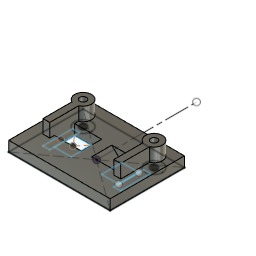
sensor_base (Autodesk Fusion 360 design; units mm, degrees)
Autodesk Fusion 360 part; units mm, degrees
sketch "Schizzo1" plane through (0, 0, 0) normal (0, 0, 1) x (1, 0, 0)
  line L0 (15, -11) -> (-15, -11)
  line L1 (-15, -11) -> (-15, 11)
  line L2 (-15, 11) -> (15, 11)
  line L3 (15, 11) -> (15, -11)
  line L4 (15, -11) -> (-15, 11) construction
  line L5 (-15, -11) -> (15, 11) construction
  circle A0 centre (-10.5, 6.5) radius 1
  line L6 (0, 0) -> (0, 29.5876)
  circle A1 centre (10.5, 6.5) radius 1
  line L7 (-4.5, -3) -> (-9.5, -3)
  line L8 (-9.5, -3) -> (-9.5, 3)
  line L9 (-9.5, 3) -> (-4.5, 3)
  line L10 (-4.5, 3) -> (-4.5, -3)
  line L11 (-4.5, -3) -> (-9.5, 3) construction
  line L12 (-9.5, -3) -> (-4.5, 3) construction
  line L13 (4.5, -3) -> (9.5, -3)
  line L14 (9.5, -3) -> (9.5, 3)
  line L15 (9.5, 3) -> (4.5, 3)
  line L16 (4.5, 3) -> (4.5, -3)
  circle A2 centre (-10.5, 6.5) radius 2.5
  circle A3 centre (10.5, 6.5) radius 2.5
  line L17 (-9.5, 4.3778) -> (-11.5, 4.3778)
  line L18 (-11.5, 4.3778) -> (-11.5, -4.3778)
  line L19 (-11.5, -4.3778) -> (-9.5, -4.3778)
  line L20 (-9.5, -4.3778) -> (-9.5, 4.3778)
  line L21 (-9.5, 4.3778) -> (-11.5, -4.3778) construction
  line L22 (-11.5, 4.3778) -> (-9.5, -4.3778) construction
  line L23 (9.5, 4.3778) -> (11.5, 4.3778)
  line L24 (11.5, -4.3778) -> (9.5, -4.3778)
  line L25 (11.5, 4.3778) -> (11.5, -4.3778)
  line L26 (9.5, -3) -> (9.5, 3)
  line L27 (9.5, -4.3778) -> (9.5, 4.3778)
  point P0 (-7, 0)
  point P1 (-10.5, 0)
  dimension "d1" = 30
  dimension "d2" = 22
  dimension "d3" = 2
  dimension "d4" = 10.5
  dimension "d6" = 4.5
  dimension "d7" = 4.5
  dimension "d8" = 5
  dimension "d9" = 6
  dimension "d10" = 5
  dimension "d11" = 5
  dimension "d12" = 2
  dimension "d13" = 8.7557
  dimension "d14" = 10.5
  constraint horizontal L0
  constraint perpendicular L0 L1
  constraint parallel L0 L2
  constraint parallel L1 L3
  constraint coincident L4 L6.start
  constraint coincident L5 L6.start
  constraint coincident L6.start origin
  constraint vertical L6
  constraint symmetric A0 L6 A1
  constraint horizontal L7
  constraint perpendicular L7 L8
  constraint parallel L7 L9
  constraint parallel L8 L10
  constraint coincident L11 P0
  constraint coincident L12 P0
  constraint symmetric L6 L7.start L13.start
  constraint symmetric L6 L7.end L13.end
  constraint symmetric L6 L8.end L14.end
  constraint symmetric L6 L9.end L15.end
  constraint concentric A0 A2
  constraint concentric A1 A3
  constraint horizontal L17
  constraint perpendicular L17 L18
  constraint parallel L17 L19
  constraint parallel L18 L20
  constraint coincident L21 P1
  constraint coincident L22 P1
  constraint symmetric L6 L17.start L23.start
  constraint symmetric L6 L17.end L23.end
  constraint symmetric L6 L18.end L24.start
  constraint symmetric L6 L19.end L24.end
  measures "d1" distance of L1.end L2.end
  measures "d2" distance of L0.end L1.end
  measures "d3" diameter of A0
  measures "d4" horizontal distance of L6.start A0.centre
  measures "d6" distance of L1 A0.centre
  measures "d7" distance of L2 A0.centre
  measures "d8" distance of L8.end L9.end
  measures "d9" distance of L7.end L8.end
  measures "d10" diameter of A2
  measures "d11" diameter of A3
  measures "d12" distance of L18.end L19.end
  measures "d13" distance of L17.end L18.end
  measures "d14" distance of L6.start P1
extrude "Estrusione1" add sketch "Schizzo1" along normal blind 3 contours L0 L1 L2 L3 | L8 A2 L18 L19 L20 | A2 L17 L18 L20 | A2 L17 L18 L20 | L14 A3 L24 L25 L26 L27 | A3 L23 L25 L27 | A3 L23 L25 L27
extrude "Estrusione2" add sketch "Schizzo1" along normal blind 4 from surface at 3 contours L8 A2 L18 L19 L20 | A2 L17 L18 L20 | A2 L17 L18 L20 | L14 A3 L24 L25 L26 L27 | A3 L23 L25 L27 | A3 L23 L25 L27
chamfer "Smusso1" distance 3 angle 45 2 edges at (-4.5, 0, 3) (4.5, 0, 3)
equation "d4 = ( 21 / 2 ) * 1 mm"
equation "d14 = ( 21 / 2 ) * 1 mm"
